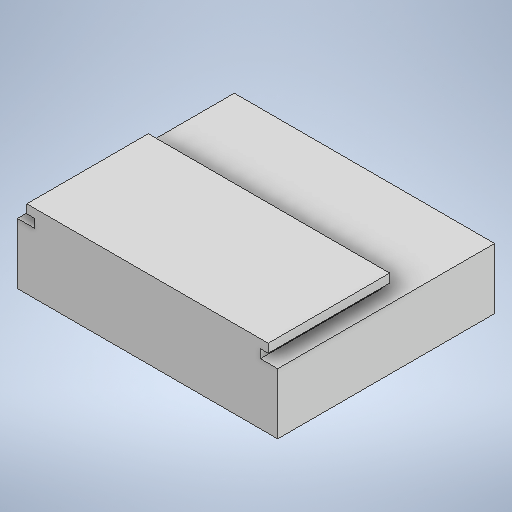
# Autodesk Inventor part: DummyModule
Saved by Autodesk Inventor 2025.3 (Build 293356000, 356)
## iProperties
Created: 2025-04-27
Part Number: DummyModule
Material: 일반
Document SubType Name: Modeling
Designer: SEON
Density: 1 g/cm^3
Appearance: 기본값
Author: SEON
Autodesk Inventor part; units mm, degrees
ref_plane "YZ Plane" through (0, 0, 0) normal (1, 0, 0) x (0, 1, 0)
ref_plane "XZ Plane" through (0, 0, 0) normal (0, 1, 0) x (-1, 0, 0)
ref_plane "XY Plane" through (0, 0, 0) normal (0, 0, 1) x (1, 0, 0)
sketch "스케치1" plane through (0, 0, 0) normal (0, 0, 1) x (1, 0, 0)
  line L0 (0, 0) -> (300, 0)
  line L1 (300, 0) -> (300, 70)
  line L2 (300, 70) -> (280, 70)
  line L3 (280, 70) -> (280, 80)
  line L4 (20, 80) -> (20, 70)
  line L5 (20, 70) -> (0, 70)
  line L6 (0, 70) -> (0, 0)
  line L7 (20, 80) -> (10.8881, 80)
  line L8 (10.8881, 80) -> (10.8881, 90)
  line L9 (10.8881, 90) -> (289.1119, 90)
  line L10 (289.1119, 90) -> (289.1119, 80)
  line L11 (289.1119, 80) -> (280, 80)
  line L12 (20, 70) -> (280, 70)
  point P0 (150, 0)
  point P1 (150, 90)
  dimension "d0" = 300
  dimension "d1" = 70
  dimension "d2" = 10
  dimension "d3" = 20
  dimension "d4" = 10
  dimension "d5" = 9.1119
  constraints: 26 end point, 8 perpendicular, 3 horizontal, 3 point on line, 2 midpoint, 1 collinear, 1 horizontal alignment, 1 vertical alignment
  measures "d0" distance of L0.start L0.end
  measures "d1" distance of L5.end L0.start
  measures "d2" distance of L4.start L4.end
  measures "d3" distance between parallel lines of L6 L4
  measures "d4" distance of L7.end L8.end
  measures "d5" distance between parallel lines of L4 L8
extrude "돌출1" add sketch "스케치1" along normal blind 250
extrude "돌출2" cut sketch "스케치1" along normal blind 110 contours L4 L7 L8 L9 L10 L11 L3 L12
